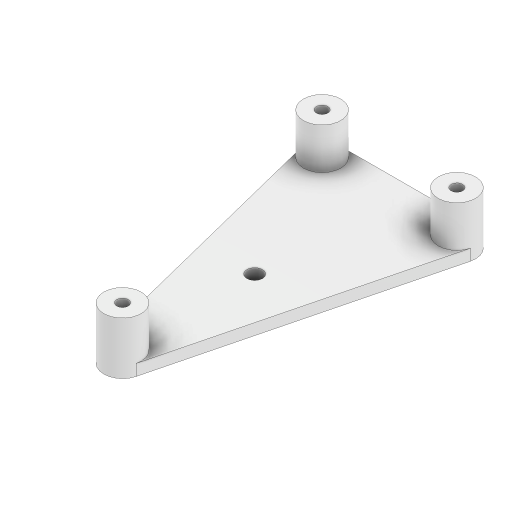
# Autodesk Inventor part: BASE_LIDAR_V3
Saved by Autodesk Inventor 2024.2 (Build 282272000, 272)
## iProperties
Created: 2024-07-17
Part Number: BASE_LIDAR_V3
Material: ABS Plastic
Document SubType Name: Modeling
Designer: jrcer
Density: 1.06 g/cm^3
Appearance: Smooth - White
Author: jrcer
Autodesk Inventor part; units mm, degrees
ref_plane "YZ Plane" through (0, 0, 0) normal (1, 0, 0) x (0, 1, 0)
ref_plane "XZ Plane" through (0, 0, 0) normal (0, 1, 0) x (-1, 0, 0)
ref_plane "XY Plane" through (0, 0, 0) normal (0, 0, 1) x (1, 0, 0)
sketch "Sketch1" plane through (0, 0, 0) normal (0, 1, 0) x (-1, 0, 0)
  circle A0 centre (0, 35.3) radius 1.55
  circle A1 centre (18, -36) radius 1.55
  circle A2 centre (-18, -36) radius 1.55
  circle A3 centre (0, 35.3) radius 5
  circle A4 centre (18, -36) radius 5
  circle A5 centre (-18, -36) radius 5
  point P0 (0, 0)
  dimension "d0" = 35.3
  dimension "d1" = 36
  dimension "d2" = 3.1
  dimension "d3" = 10
  dimension "d4" = 36
  dimension "d5" = 18
  constraints: 6 centre point, 4 equal radius, 3 coincident, 1 horizontal alignment, 1 vertical alignment
  measures "d0" distance of A0.centre point (0, 0)
  measures "d1" vertical distance of A2.centre point (0, 0)
  measures "d2" diameter of A0
  measures "d3" diameter of A3
  measures "d4" distance of A2.centre A1.centre
  measures "d5" horizontal distance of point (0, 0) A2.centre
extrude "Extrusion1" add sketch "Sketch1" along normal blind 11
sketch "Sketch2" plane through (0, 0, 35.3) normal (0, -1, 0) x (1, 0, 0)
  circle A0 centre (0, 0) radius 5 projected
  circle A1 centre (0, 0) radius 1.55 projected
  circle A2 centre (-18, -71.3) radius 1.55 projected
  circle A3 centre (-18, -71.3) radius 5 projected
  circle A4 centre (18, -71.3) radius 1.55 projected
  circle A5 centre (18, -71.3) radius 5 projected
  line L0 (-22.8479, -70.0761) -> (-4.8479, 1.2239)
  line L1 (22.8479, -70.0761) -> (4.8479, 1.2239)
  line L2 (-18, -76.3) -> (18, -76.3)
  circle A6 centre (0, -35.3) radius 2.1
  dimension "d8" = 4.2
  constraints: 6 end point, 6 point on circle, 5 tangent, 1 centre point, 1 coincident, 1 horizontal
  measures "d8" diameter of A6
extrude "Extrusion2" add sketch "Sketch2" along normal blind 3
equation "\"d5\" = 0.5 * d4"
body "Solid1"
